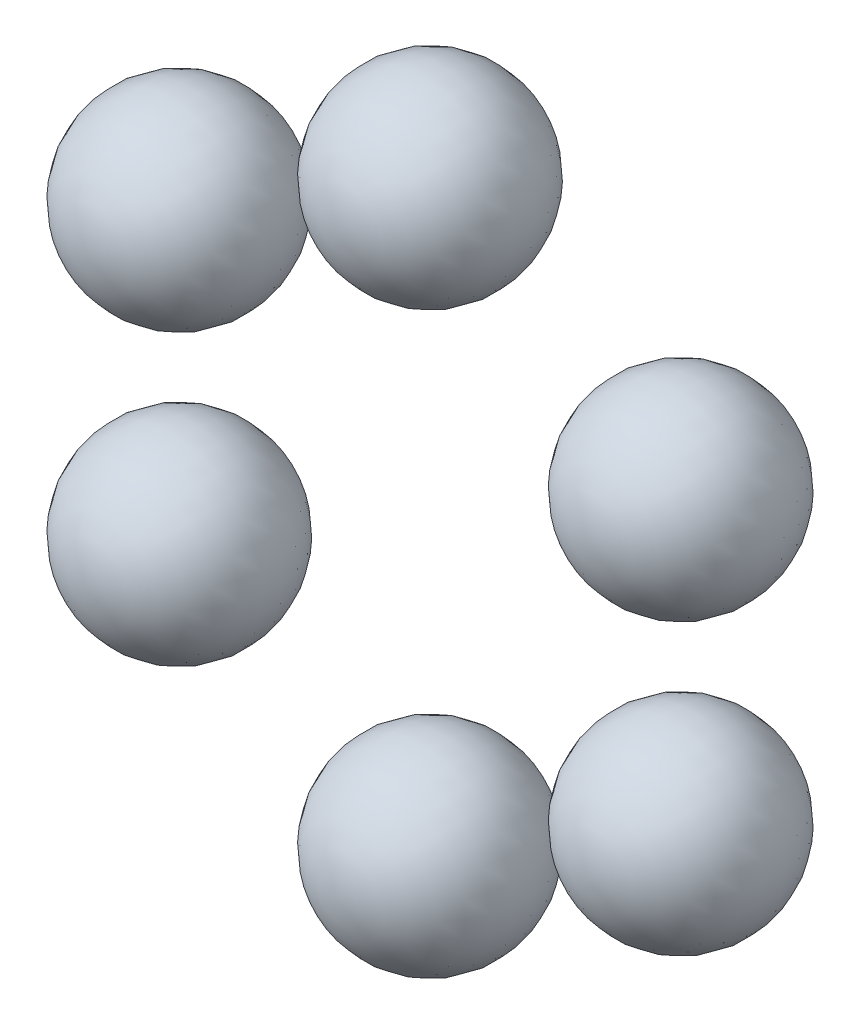
# Autodesk Inventor part: balines
Saved by Autodesk Inventor 2021 (Build 250183000, 183)
## iProperties
Created: 2021-04-24
Part Number: balines
Material: Genérico
Document SubType Name: Modeling
Designer: j2seb
Density: 1 g/cm^3
Appearance: Valor por defecto
Author: j2seb
Autodesk Inventor part; units mm, degrees
ref_plane "YZ Plane" through (0, 0, 0) normal (1, 0, 0) x (0, 1, 0)
ref_plane "XZ Plane" through (0, 0, 0) normal (0, 1, 0) x (-1, 0, 0)
ref_plane "XY Plane" through (0, 0, 0) normal (0, 0, 1) x (1, 0, 0)
sketch "Boceto2" plane through (0, 0, 0) normal (0, 0, 1) x (1, 0, 0)
  circle A0 centre (0, -17.75) radius 5.75
  circle A1 centre (0, 0) radius 12 construction
  circle A2 centre (0, 0) radius 23.5 construction
  line L0 (0, 0) -> (0, -23.5)
  point P0 (0, -12)
  dimension "d_out" = 47
  dimension "d_in" = 24
  constraints: 2 coincident, 2 end point, 2 vertical alignment, 1 centre point, 6 other
  measures "d_in" diameter of A1
revolve "Revolución1" add sketch "Boceto2" angle 360 about axis through (0, 0, 0) along (0, -1, 0) picked at (0.8316, -16.0231) contours L0 A0
pattern_circular "Patrón circular1" count 6 over 360 about axis through (0, 0, -10) along (0, 0, 1) of "Revolución1"
